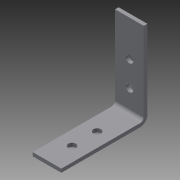
# Autodesk Inventor part: Gusset 4
Saved by Autodesk Inventor 2013 (Build 170138000, 138)
## iProperties
Created: 2013-01-31
Part Number: Gusset 4
Material: Generic
Document SubType Name: Sheet Metal
Designer: actoennies
Density: 1 g/cm^3
Sheet Metal Rule: Default
Mass: 11.4141 g
Surface Area: 85.5543 cm^2
Volume: 11.4141 cm^3
Author: actoennies
Autodesk Inventor part; units mm, degrees
ref_plane "YZ Plane" through (0, 0, 0) normal (1, 0, 0) x (0, 1, 0)
ref_plane "XZ Plane" through (0, 0, 0) normal (0, 1, 0) x (-1, 0, 0)
ref_plane "XY Plane" through (0, 0, 0) normal (0, 0, 1) x (1, 0, 0)
sketch "Sketch1" plane through (0, 0, 0) normal (0, 0, 1) x (1, 0, 0)
  line L0 (0, 0) -> (0, 76.2)
  line L1 (0, 76.2) -> (25.4, 76.2)
  line L2 (25.4, 76.2) -> (25.4, 0)
  line L3 (25.4, 0) -> (0, 0)
  circle A0 centre (12.7, 22.225) radius 3.3782
  circle A1 centre (12.7, 44.45) radius 3.3782
  dimension "d0" = 76.2
  dimension "d1" = 25.4
  dimension "d3" = 6.7564
  dimension "d4" = 22.225
  dimension "d8" = 6.7564
  measures "d0" distance of L0.start L0.end
  measures "d1" distance of L0.end L1.end
  measures "d3" diameter of A0
  measures "d4" distance from line of L3 A0.centre
  measures "d8" diameter of A1
extrude "Plate1" add sketch "Sketch1" along normal blind 3.175
sketch "Sketch2" plane through (25.4, 3.175, 0) normal (0, -1, 0) x (1, 0, 0)
  line L0 (-25.4, 0) -> (0, 0)
  line L1 (0, 0) -> (0, 76.2)
  line L2 (0, 76.2) -> (-25.4, 76.2)
  line L3 (-25.4, 76.2) -> (-25.4, 0)
  constraints: 6 end point, 1 horizontal, 1 perpendicular, 1 vertical
edge flange "Flange1" height 76.2 angle 90 thickness 3.175 bend radius 3.175 thickness toward (0, -1, 0) relief straight relief width 3.175 relief depth 1.5875 edges at (12.7, 0, 3.175) wall of the first edge with corners at (0, 3.175, 0) (25.4, 3.175, 0) (25.4, 3.175, 76.2) (0, 3.175, 76.2)
bend "Bend1"
corner "Corner1"
sketch "Sketch3" plane through (0, 3.175, 76.2) normal (0, 1, 0) x (1, 0, 0)
  line L0 (0, 0) -> (25.4, 0) projected
  circle A0 centre (12.7, 44.45) radius 3.3782
  circle A1 centre (12.7, 22.225) radius 3.3782
  line L1 (0, 76.2) -> (0, 73.025) projected
  dimension "d21" = 6.7564
  dimension "d22" = 6.7564
  dimension "d23" = 12.7
  dimension "d24" = 22.225
  dimension "d25" = 22.225
  constraints: 2 centre point
  measures "d21" diameter of A0
  measures "d22" diameter of A1
  measures "d23" distance from line of L1 A0.centre
  measures "d24" distance from line of L0 A1.centre
  measures "d25" distance of A1.centre A0.centre
extrude "Cut1" cut sketch "Sketch3" against normal blind 3.175
equation "\"d26\" = Thickness"
equation "\"d11\" = BendReliefWidth"
equation "\"d12\" = BendReliefDepth"
equation "\"d13\" = MinimumRemnant"
equation "\"d14\" = BendRadius"
equation "\"d17\" = BendRadius"
equation "\"d18\" = CornerReliefSize"
equation "\"d19\" = GapSize"
equation "\"d20\" = JacobiRadiusSize"
equation "\"BendRadius\" = Thickness"
equation "\"BendReliefWidth\" = Thickness"
equation "\"BendReliefDepth\" = 0.5 * Thickness"
equation "\"CornerReliefSize\" = 4 * Thickness"
equation "\"MinimumRemnant\" = 2 * Thickness"
equation "\"TransitionRadius\" = BendRadius"
equation "\"JacobiRadiusSize\" = BendRadius"
equation "\"GapSize\" = Thickness"
equation "\"d10\" = BendRadius"
equation "\"Thickness\" = 3.175"
body "Solid1"
